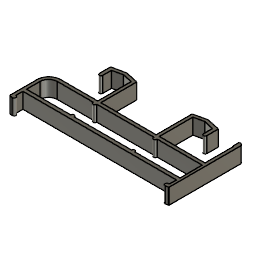
RielDoble (Autodesk Fusion 360 design; units mm, degrees)
part number: 2025-12-26-21-56-54-991
Autodesk Fusion 360 part; units mm, degrees
sketch "Boceto1" plane through (0, 0, 0) normal (0, 0, 1) x (1, 0, 0)
  line L0 (2, 0) -> (2, 8.65)
  line L1 (101.8, 16.3) -> (101.85, 16.3)
  arc A0 (7.5, 14.15) -> (2, 8.65) centre (7.5, 8.65) ccw
  arc A1 (7.5, 16.3) -> (0, 8.8) centre (7.5, 8.8) ccw
  line L2 (2, -2.3) -> (2, -6.9)
  line L3 (2.3, -2.3) -> (2, -2.3)
  line L4 (2.3, -2.3) -> (100.158, -2.3)
  line L5 (101.8, 3.1911) -> (101.8, -8.6712)
  line L6 (101.8, 3.1911) -> (101.8, 37.4)
  line L7 (99.8001, 16.3) -> (99.8001, 34.1999)
  line L8 (100.158, 14.15) -> (100.158, 0)
  line L9 (100.158, -2.3) -> (100.158, -6.3898)
  arc A2 (2, -9.2) -> (2, -6.9) centre (2.15, -8.05) ccw
  arc A3 (2, -9.2) -> (0.4131, -9.0314) centre (-2.3285, -42.3855) ccw
  arc A4 (0, -8.5829) -> (0.4131, -9.0314) centre (0.45, -8.5829) ccw
  arc A5 (99.6517, -6.8897) -> (99.7844, -9.1637) centre (99.6375, -8.0314) ccw
  arc A6 (99.7844, -9.1637) -> (101.6373, -8.8677) centre (95.6739, 22.5158) ccw
  arc A7 (101.6373, -8.8677) -> (101.8, -8.6712) centre (101.6, -8.6712) ccw
  arc A8 (30.5215, 14.15) -> (32.7096, 14.15) centre (31.6155, 13.9852) ccw
  arc A9 (32.6, 0) -> (30.251, 0) centre (31.4255, -0.0135) ccw
  arc A10 (71.3285, -0.0135) -> (69.1583, 0) centre (70.2436, 0.0214) ccw
  arc A11 (69.2318, 14.15) -> (71.3896, 14.15) centre (70.3107, 13.9445) ccw
  line L10 (30.5215, 14.15) -> (7.5, 14.15)
  line L11 (100.158, 14.15) -> (71.3896, 14.15)
  line L12 (69.2318, 14.15) -> (32.7096, 14.15)
  line L13 (71.3289, 0) -> (100.158, 0)
  line L14 (2, 0) -> (30.251, 0)
  line L15 (32.6, 0) -> (69.1583, 0)
  line L16 (31.2519, 16.3) -> (31.2519, 37.68)
  line L17 (33.2, 16.3) -> (33.2, 39.3)
  line L18 (31.2519, 37.68) -> (25, 39)
  line L19 (25, 39) -> (18.7, 37.6)
  line L20 (18.7, 37.6) -> (18.7, 32)
  line L21 (16.478, 32) -> (16.478, 39.3)
  line L22 (16.478, 39.3) -> (25, 41.1)
  line L23 (25, 41.1) -> (33.2, 39.3)
  arc A12 (16.478, 32) -> (18.7, 32) centre (17.589, 32) ccw
  line L24 (31.2519, 16.3) -> (7.5, 16.3)
  line L25 (68.6, 16.3) -> (68.6, 39.3094)
  line L26 (68.6, 39.3094) -> (76.8919, 41.1826)
  line L27 (76.8919, 41.1826) -> (85.3377, 39.3705)
  line L28 (85.3377, 39.3705) -> (85.3377, 31.9)
  line L29 (83.2, 31.9) -> (83.2, 37.6)
  line L30 (83.2, 37.6) -> (76.8919, 39.1275)
  line L31 (76.8919, 39.1275) -> (70.6157, 37.7097)
  line L32 (70.6157, 37.7097) -> (70.6157, 16.3)
  line L33 (99.9, 16.3) -> (70.6157, 16.3)
  line L34 (68.6, 16.3) -> (33.2, 16.3)
  arc A13 (83.2, 31.9) -> (85.3377, 31.9) centre (84.2689, 31.9) ccw
  arc A14 (101.8, 37.4) -> (99.8001, 38.7495) centre (99.8323, 36.6406) ccw
  line L35 (99.4, 38.4) -> (99.4, 34.6554)
  arc A15 (99.8001, 38.7495) -> (99.4, 38.4) centre (99.8537, 38.2844) ccw
  arc A16 (99.4429, 34.5504) -> (99.8001, 34.3936) centre (99.8167, 34.9167) ccw
  line L36 (99.8001, 34.1999) -> (99.8001, 34.3936)
  arc A17 (99.4, 34.6554) -> (99.4429, 34.5504) centre (99.55, 34.6554) ccw
  arc A18 (99.6517, -6.8897) -> (100.158, -6.3898) centre (99.658, -6.3898) ccw
  line L37 (0, 8.8) -> (0, -8.5829)
  dimension "d1" = 101.85
  dimension "d3" = 5.5
  dimension "d4" = 7.5
  dimension "d5" = 0.45
  dimension "d6" = 0.2
  dimension "d7" = 0.15
  dimension "d8" = 0.5
  constraint horizontal L14
  constraint perpendicular L0 L33
  constraint parallel L1 L33
  constraint tangent A0 L11
  constraint tangent L0 A0
  constraint tangent A1 L33
  constraint perpendicular L8 L14
  constraint perpendicular L2 L14
  constraint perpendicular L2 L4
  constraint perpendicular L4 L5
  constraint perpendicular L6 L14
  constraint perpendicular L7 L33
  constraint coincident L7.start L33
  constraint collinear L8 L9
  constraint tangent A2 A3
  constraint tangent A3 A4
  constraint tangent A5 A6
  constraint tangent A6 A7
  constraint tangent L5 A7
  constraint coincident A8.start L11
  constraint coincident A9.start L14
  constraint coincident A11.start L11
  constraint collinear L10 L11
  constraint collinear L11 L12
  constraint coincident A10 L13.start
  constraint collinear L13 L14
  constraint collinear L14 L15
  constraint coincident L16.start L33
  constraint perpendicular L16 L33
  constraint perpendicular L17 L33
  constraint vertical L20
  constraint collinear L24 L33
  constraint coincident L25.start L33
  constraint perpendicular L25 L33
  constraint parallel L25 L28
  constraint parallel L26 L31
  constraint perpendicular L32 L33
  constraint collinear L33 L34
  constraint parallel L7 L35
  constraint parallel L7 L36
  constraint tangent L35 A17
  constraint tangent A16 A17
  constraint coincident L6 L1.start
  constraint tangent A5 A18
  constraint tangent L9 A18
  constraint tangent A4 L37
  measures "d1" distance of origin L5.start
  measures "d3" radius of A0
  measures "d4" radius of A1
  measures "d5" radius of A4
  measures "d6" radius of A7
  measures "d7" radius of A17
  measures "d8" radius of A18
extrude "Extruir1" add sketch "Boceto1" along normal blind 10
equation "L = 10 mm"
equation "d10 = L"
